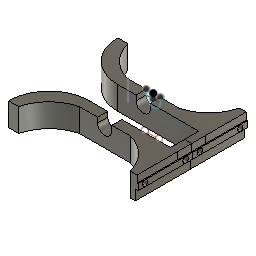
Rubbermade 2020 Holder (Autodesk Fusion 360 design; units mm, degrees)
Autodesk Fusion 360 part; units mm, degrees
sketch "Sketch1" plane through (0, 0, 0) normal (0, 0, 1) x (1, 0, 0)
  line L0 (-9.5216, -0.1214) -> (70.4784, -0.1214)
  line L1 (77.4784, -0.1214) -> (77.4784, 39.8786)
  line L2 (-49.5216, 39.8786) -> (-39.5216, 39.8786)
  line L3 (77.4784, 39.8786) -> (70.4784, 39.8786)
  line L4 (-9.5216, 9.8786) -> (40.4784, 9.8786)
  line L5 (70.4784, 39.8786) -> (40.4784, 39.8786) construction
  line L6 (-9.5216, 39.9434) -> (-9.5216, 9.8786) construction
  line L7 (40.4784, 39.8786) -> (40.4784, 9.8786) construction
  arc A0 (-39.5863, 39.8786) -> (-9.5216, 9.8786) centre (-9.5216, 39.9434) ccw
  arc A1 (40.4784, 9.8786) -> (70.4784, 39.8786) centre (40.4784, 39.8786) ccw
  line L8 (77.4784, -0.1214) -> (77.4784, -14.1214)
  line L9 (77.4784, -14.1214) -> (70.4784, -14.1214)
  line L10 (70.4784, -14.1214) -> (70.4784, -0.1214)
  arc A2 (-49.5216, 39.8786) -> (-9.5216, -0.1214) centre (-9.5216, 39.8786) ccw
  line L11 (0, 0) -> (-49.5216, -0.0008) construction
  line L12 (-49.5216, -0.0008) -> (-49.5216, 39.8786) construction
  arc A3 (40.4784, 9.8786) -> (70.4784, 39.8786) centre (31.1328, 49.2241) ccw
  arc A4 (-39.5863, 39.8786) -> (-9.5216, 9.8786) centre (0.3476, 49.8338) ccw
  point P0 (70.4784, 39.8786)
  point P1 (40.4784, 9.8786)
  point P2 (-9.5216, 9.8786)
  point P3 (-39.5216, 39.9434)
  point P4 (-28.7716, 20.7495)
  point P5 (-30.7577, 18.6614)
  point P6 (59.7284, 20.6286)
  point P7 (61.6916, 18.6654)
  dimension "d3" = 40
  dimension "d4" = 10
  dimension "d7" = 10
  dimension "d9" = 30
  dimension "d10" = 30
  dimension "d11" = 14
  dimension "d37" = 7
  dimension "d38" = 120
  dimension "d44" = 20.75
  dimension "d45" = 20.75
  dimension "d46" = 4.7564
  dimension "d47" = 20.75
  dimension "d48" = 17.75
  dimension "d67" = 30
  dimension "d68" = 80
  dimension "d69" = 50
  dimension "d70" = 14
  dimension "d71" = 14
  dimension "d72" = 30
  constraint perpendicular L4 L6
  constraint perpendicular L4 L7
  constraint coincident L6.start A0.centre
  constraint coincident L5.end L7.start
  constraint tangent L4 A1
  constraint coincident P0 L3.end
  constraint coincident P1 L4.end
  constraint coincident P2 L4.start
  constraint coincident L2 A0.start
  constraint perpendicular L1 L3
  constraint perpendicular L5 L7
  constraint equal L3 L9
  constraint tangent L0 A2
  constraint midpoint A0 P5
  constraint coincident L11.start origin
  constraint perpendicular L2 L12
  constraint coincident P6 A3
  constraint midpoint A1 P7
  constraint parallel L8 L10
  constraint parallel L1 L6
  constraint parallel L0 L2
  constraint coincident P4 A4
  measures "d3" distance of L1.start L1.end
  measures "d4" distance of L2.start L2.end
  measures "d7" distance of L0 L4
  measures "d9" distance of L6.start P3
  measures "d10" distance of P0 L5.end
  measures "d11" distance of L1.start L8.end
  measures "d37" distance of L1.end P0
  measures "d38" distance of L2.start L10
  measures "d44" distance of P4 L11
  measures "d45" distance of P4 L12
  measures "d47" distance of L0 P6
  measures "d48" distance of L1 P6
  measures "d67" vertical distance of P1 P0
  measures "d68" distance of L0.end L0.start
  measures "d69" distance of P2 P1
  measures "d70" vertical distance of L1.start L8.end
  measures "d71" distance of L9.end L0.end
  measures "d72" distance of L2 L4
extrude "Extrude1" add sketch "Sketch1" along normal blind 20 makes body 1
sketch "Sketch2" plane through (77.4784, 0, 0) normal (1, 0, 0) x (0, 1, 0)
  line L0 (-14.1214, 0) -> (-0.1214, 0)
  line L1 (39.8786, 0) -> (39.8786, 20)
  line L2 (-0.1214, 20) -> (-14.1214, 20)
  line L3 (-14.1214, 20) -> (-14.1214, 0)
  line L4 (-14.1214, 13) -> (39.8786, 13)
  line L5 (39.8786, 13) -> (39.8786, 7)
  line L6 (39.8786, 7) -> (-14.1214, 7)
  line L7 (-14.1214, 7) -> (-14.1214, 13)
  circle A0 centre (-7.1214, 10) radius 2.75
  circle A1 centre (-7.1214, 10) radius 5
  circle A2 centre (32.8786, 10) radius 2.75
  circle A3 centre (32.8786, 10) radius 5
  line L8 (-0.1214, 0) -> (-0.1214, 20)
  line L9 (-0.1214, 0) -> (39.8786, 0)
  line L10 (39.8786, 20) -> (-0.1214, 20)
  line L11 (-0.1214, 20) -> (-0.1214, 0)
  dimension "d15" = 6
  dimension "d16" = 7
  dimension "d19" = 5.5
  dimension "d20" = 10
  dimension "d21" = 5.5
  dimension "d22" = 10
  dimension "d23" = 7
  dimension "d24" = 7
  dimension "d25" = 10
  dimension "d26" = 10
  constraint perpendicular L4 L5
  constraint parallel L4 L6
  constraint parallel L5 L7
  constraint coincident L1 L4.end
  constraint perpendicular L1 L4
  constraint coincident L3 L4.start
  constraint concentric A0 A1
  constraint concentric A2 A3
  measures "d15" distance of L4.start L6.end
  measures "d16" distance of L0 L6
  measures "d19" diameter of A0
  measures "d20" diameter of A1
  measures "d21" diameter of A2
  measures "d22" diameter of A3
  measures "d23" distance of L7 A0.centre
  measures "d24" distance of L1 A2.centre
  measures "d25" distance of L2 A0.centre
  measures "d26" distance of L2 A2.centre
extrude "Extrude2" add sketch "Sketch2" along normal blind 1 contours L3 L4 L6 L7 A1 | L4 L6 A3 L8 L11 | L4 L6 A1 L8 L11 | L4 L6 A1 | L4 L6 A3 | L1 L4 L5 L6 A3 | A0 | A2 bodies 1
extrude "Extrude3" cut sketch "Sketch2" against normal blind 20 from surface at 1 contours A0 | A2 bodies 1
extrude "Extrude4" cut sketch "Sketch2" against normal blind 25 from surface at -3 contours L4 L6 A1 | L6 A1 | L4 L6 A3 | L6 A3 | L4 A1 | L4 A3 bodies 1
sketch "Sketch3" plane through (0, 9.8786, 0) normal (0, 1, 0) x (1, 0, 0)
  line L0 (40.4784, 0) -> (-9.5216, 0)
  line L1 (-9.5216, -20) -> (40.4784, -20)
  line L2 (40.4784, -20) -> (40.4784, 0)
  line L3 (13.9164, 16.5) -> (20.9164, 16.5) construction
  line L4 (13.9164, 16.5) -> (6.9164, 16.5) construction
  line L5 (15.4449, -15) -> (22.4449, -15) construction
  line L6 (15.4449, -15) -> (8.4449, -15) construction
  line L7 (22.4449, -15) -> (22.4449, -20)
  line L8 (8.4449, -15) -> (8.4449, -20)
  arc A0 (22.4449, -15) -> (8.4449, -15) centre (15.4449, -15) ccw
  line L9 (-9.5216, 0) -> (-9.5216, -20)
  point P0 (15.4784, -20)
  dimension "d56" = 14
  dimension "d57" = 5
  constraint horizontal L3
  constraint parallel L3 L4
  constraint midpoint L1 P0
  constraint coincident L5.start L6.start
  constraint horizontal L5
  constraint parallel L5 L6
  constraint coincident L1 L7.end
  constraint coincident L1 L8.end
  constraint tangent L7 A0
  constraint tangent L8 A0
  measures "d56" diameter of A0
  measures "d57" distance of L1 L5.start
extrude "Extrude7" cut sketch "Sketch3" against normal up to surface (10 mm away) contours L1 L7 L8 A0 bodies 1
extrude "Extrude8" add 1 faces at (73.7992, 23.088, 0) along direction (0, 0, -1) blind 3 on bodies 1 bodies 1
mirror "Mirror1" about plane through (77.4784, -14.1214, 0) normal (0, -1, 0) of bodies 1 makes body 2
extrude "Extrude9" cut 2 faces at (77.4784, -18.7881, 0.3333) (77.4784, -41.4548, 3.6667) along direction (-1, 0, 0) blind 1.62 on bodies 2 bodies 2
extrude "Extrude10" cut 2 faces at (77.4784, -9.4548, 0.3333) (77.4784, 13.2119, 3.6667) along direction (-1, 0, 0) blind 1.62 on bodies 1 bodies 1
equation "d48 = 20.75 mm - 3 mm"
